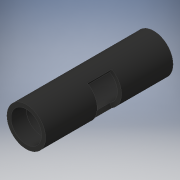
# Autodesk Inventor part: DPLX_P033_SG_Viton rubber Cover
Saved by Autodesk Inventor 2018 (Build 220112000, 112)
## iProperties
Created: 2017-12-13
Part Number: DPLX_P033_SG_Viton rubber Cover
Material: Rubber, Silicone
Document SubType Name: Modeling
Designer: Pierce
Density: 1.25 g/cm^3
Appearance: Rubber - Black
Mass: 31.0136 g
Surface Area: 165.13 cm^2
Volume: 24.8109 cm^3
Author: Pierce
Autodesk Inventor part; units mm, degrees
ref_plane "YZ Plane" through (0, 0, 0) normal (1, 0, 0) x (0, 1, 0)
ref_plane "XZ Plane" through (0, 0, 0) normal (0, 1, 0) x (-1, 0, 0)
ref_plane "XY Plane" through (0, 0, 0) normal (0, 0, 1) x (1, 0, 0)
sketch "Sketch1" plane through (0, 0, 0) normal (0, 0, 1) x (1, 0, 0)
  circle A0 centre (0, 0) radius 12
  circle A1 centre (0, 0) radius 15.175
  dimension "d0" = 24
  dimension "d1" = 3.175
  constraints: 2 centre point, 1 coincident
  measures "d0" diameter of A0
  measures "d1" radial gap between concentric circles of A0 A1
extrude "Extrusion1" add sketch "Sketch1" along normal mid plane 100
sketch "Sketch2" plane through (0, 0, 0) normal (0, 1, 0) x (-1, 0, 0)
  line L0 (15.175, -50) -> (15.175, 50) projected
  line L1 (-12, -50) -> (-12, 50) projected
  line L2 (-15.175, -50) -> (-15.175, 50) projected
  line L3 (15.175, 12.7) -> (15.175, -12.7)
  line L4 (0, -70) -> (0, 70) projected
  line L5 (-12, -50) -> (-12, 50) projected
  line L6 (-12, -9.525) -> (-15.175, -9.525)
  line L7 (-15.175, -9.525) -> (-15.175, 9.525)
  line L8 (-15.175, 9.525) -> (-12, 9.525)
  line L9 (-12, 9.525) -> (-12, -9.525)
  point P0 (0, 0)
  point P1 (12, 0)
  point P2 (-12, 0)
  dimension "d6" = 19.05
  constraints: 10 end point, 3 point on line, 2 horizontal alignment, 2 parallel, 1 horizontal, 1 midpoint, 1 perpendicular
  measures "d6" distance between parallel lines of L8 L6
revolve "Revolution1" cut sketch "Sketch2" angle 120 mid plane about axis through (0, 0, -10) along (0, 0, 1)
sketch "Sketch4" plane through (0, 0, 0) normal (0, 0, 1) x (1, 0, 0)
  arc A0 (6.8593, 9.8463) -> (6.8593, -9.8463) centre (0, 0) ccw
  arc A1 (6.8593, 9.8636) -> (6.8593, -9.8636) centre (0, 0) ccw
  line L0 (6.8593, 9.8636) -> (6.8593, 9.8463)
  line L1 (6.8593, -9.8463) -> (6.8593, -9.8636)
  dimension "d9" = 24.0284
  constraints: 4 end point, 4 point on circle, 2 centre point, 2 coincident
  measures "d9" diameter of A1
extrude "Extrusion2" cut sketch "Sketch4" along normal mid plane 76.2
body "Solid1"
